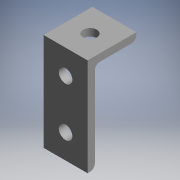
# Autodesk Inventor part: 20-4176 Aluminum
Saved by Autodesk Inventor 2017.3 (Build 213256000, 256)
## iProperties
Part Number: 20-4176 Aluminum
Material: Generic
Catalog Web Link: www.cadenas.de
Description: 25-4176, 40-4376, 20-4176, 30-4376, 45-4376, 25-4176-Black, 40-4376-Black, 20-4176-Black, 30-4376-Black, 45-4376-Black-3 Hole Inside Corner Bracket
Vendor: 8020
Document SubType Name: Modeling
Designer: partserver
Manufacturer: 8020
Mass: 2.84403 g
Surface Area: 24.6546 cm^2
Volume: 2.84403 cm^3
Density: 1 g/cm^3
Appearance: PSOLRGB-191-191-191
Category: PARTsolutions
Company: 8020
Title: 20-4176
Author: Cadenas PARTsolutions
Comments: 3 Hole Inside Corner Bracket
PSOL_IDENT_0: {$CADENAS_DATA\23d-libs\8020\metric\joining_plates\25_4176.prj},266 {VTYP=3D},{NB=20-4176},{LINA=20-
PSOL_IDENT_1: 4176},{NN=25-4176, 40-4376, 20-4176, 30-4376, 45-4376, 25-4176-Black, 40-4376-Black, 20-4176-Black,
PSOL_IDENT_2: 30-4376-Black, 45-4376-Black},{DATE=31.07.2020 09:21:28},{GEOMDATE=09.01.2019 19:08:43},{VERSION=},{
PSOL_IDENT_3: LINEID=30},{WBVAR=},{WBNUMERIC=}  {NB=20-4176},{LINA=20-4176},{KT=DUMMY},{PN=20-4176},{SERIES=20},{M
PSOL_IDENT_4: ATERIAL=Aluminum},{GRADE=6105-T5},{FINISH=Clear Anodize},{A=18.00},{B=40.00},{C=20.00},{D=20.00},{E=
PSOL_IDENT_5: 10.00},{F=5.56},{T=3.00},{W=.007},{A1=10.000},{A2=30.000},{R=2.000},{COLOR=.75,.75,.75}
NB: 20-4176
NN: 25-4176, 40-4376, 20-4176, 30-4376, 45-4376, 25-4176-Black, 40-4376-Black, 20-4176-Black, 30-4376-Black, 45-4376-Black
NT: 3 Hole Inside Corner Bracket
NBSYN: $PN.
LINA: 20-4176
CATALOG: 80/20
PN: 20-4176
SERIES: 20
MATERIAL: Aluminum
GRADE: 6105-T5
FINISH: Clear Anodize
A: 18
B: 40
C: 20
D: 20
E: 10
F: 5.56
T: 3
W: .007
SUPPLIER: 8020
ARTICLENO: 20-4176
BOMINFO: 20-4176
CREATOR: CADENAS GmbH
Autodesk Inventor part; units mm, degrees
ref_plane "YZ Plane" through (0, 0, 0) normal (1, 0, 0) x (0, 1, 0)
ref_plane "XZ Plane" through (0, 0, 0) normal (0, 1, 0) x (-1, 0, 0)
ref_plane "XY Plane" through (0, 0, 0) normal (0, 0, 1) x (1, 0, 0)
sketch "Sketch_1" plane through (0, 0, 0) normal (1, 0, 0) x (0, 1, 0)
  line L0 (1, 40) -> (0, 40)
  line L1 (0, 40) -> (0, 0)
  line L2 (0, 0) -> (20, 0)
  line L3 (20, 0) -> (20, 1)
  arc A0 (20, 1) -> (18, 3) centre (18, 1) ccw
  line L4 (18, 3) -> (5, 3)
  arc A1 (3, 5) -> (5, 3) centre (5, 5) ccw
  line L5 (3, 5) -> (3, 38)
  arc A2 (3, 38) -> (1, 40) centre (1, 38) ccw
  constraints: 12 end point, 6 point on circle, 3 centre point
extrude "Extrusion1" add sketch "Sketch_1" along normal mid plane 18
sketch "Sketch2" plane through (9, 20, 0) normal (0, 0, -1) x (-1, 0, 0)
  point P0 (9, -10)
hole "Hole1" at (0, 10, 0) direction (0, 0, 1) diameter 5.56 depth 3
sketch "Sketch3" plane through (-9, 0, 0) normal (0, -1, 0) x (1, 0, 0)
  point P0 (9, 10)
hole "Hole2" at (0, 0, 10) direction (0, 1, 0) diameter 5.56 depth 3
sketch "Sketch4" plane through (-9, 0, 0) normal (0, -1, 0) x (1, 0, 0)
  point P0 (9, 30)
hole "Hole3" at (0, 0, 30) direction (0, 1, 0) diameter 5.56 depth 3
body "Solid1"
